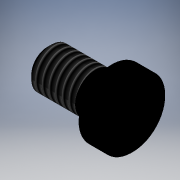
# Autodesk Inventor part: 25-2750-6
Saved by Autodesk Inventor 2017.3 (Build 213256000, 256)
## iProperties
Part Number: 25-2750-6
Material: Generic
Catalog Web Link: www.cadenas.de
Description: 25-2750_bolt-Socket Head Cap Screws
Vendor: 8020
Document SubType Name: Modeling
Designer: partserver
Manufacturer: 8020
Mass: 0.502109 g
Surface Area: 4.42769 cm^2
Volume: 0.502109 cm^3
Density: 1 g/cm^3
Appearance: PSOLRGB-0-0-0
Category: PARTsolutions
Company: 8020
Title: 25-2750-6
Author: Cadenas PARTsolutions
Comments: Socket Head Cap Screws
PSOL_IDENT_0: {$CADENAS_DATA\23d-libs\8020\metric\linear_motion\25_2750_bolt.prj},164 {VTYP=3D},{NB=25-2750-6},{LI
PSOL_IDENT_1: NA=25-2750-6},{NN=25-2750_bolt},{DATE=31.07.2020 09:21:29},{GEOMDATE=15.03.2012 10:20:00},{VERSION=}
PSOL_IDENT_2: ,{LINEID=60},{WBVAR=},{WBNUMERIC=}  {NB=25-2750-6},{LINA=25-2750-6},{KT=DUMMY},{PN=25-2750-6},{THRD=
PSOL_IDENT_3: M6 x 1.00},{THRD1=6.0000},{FIN=Black Zinc},{L=9.525},{TT=UNC},{A=10.000},{H=3.226},{J=3.17500},{T=1.
PSOL_IDENT_4: 613},{TH=6.0000},{NT=25-3204},{NO=1}
NB: 25-2750-6
NN: 25-2750_bolt
NT: 25-3204
NBSYN: $PN.
LINA: 25-2750-6
CATALOG: 80/20
PN: 25-2750-6
THRD: M6 x 1.00
FIN: Black Zinc
L: 9.525
H: 3.226
TH: 6
NO: 1
SUPPLIER: 8020
ARTICLENO: 25-2750-6
BOMINFO: 25-2750-6
CREATOR: CADENAS GmbH
Autodesk Inventor part; units mm, degrees
ref_plane "YZ Plane" through (0, 0, 0) normal (1, 0, 0) x (0, 1, 0)
ref_plane "XZ Plane" through (0, 0, 0) normal (0, 1, 0) x (-1, 0, 0)
ref_plane "XY Plane" through (0, 0, 0) normal (0, 0, 1) x (1, 0, 0)
sketch "Sketch_1" plane through (0, 0, 0) normal (0, 0, 1) x (1, 0, 0)
  line L0 (9.525, 0) -> (-3.226, 0)
  line L1 (-3.226, 0) -> (-3.226, 4.8476)
  line L2 (-3.226, 4.8476) -> (-3.0736, 5)
  line L3 (-3.0736, 5) -> (-0.254, 5)
  arc A0 (0, 4.746) -> (-0.254, 5) centre (-0.254, 4.746) ccw
  line L4 (0, 4.746) -> (0, 3.0762)
  arc A1 (0, 3.0762) -> (0.0762, 3) centre (0.0762, 3.0762) ccw
  line L5 (0.0762, 3) -> (8.9115, 3)
  line L6 (8.9115, 3) -> (9.525, 2.3865)
  line L7 (9.525, 2.3865) -> (9.525, 0)
  line L8 (9.525, 0) -> (-3.226, 0)
  constraints: 18 end point, 4 point on circle, 2 centre point
revolve "Revolution1" add sketch "Sketch_1" angle 360 about axis through (9.525, 0, 0) along (1, 0, 0)
thread "Thread1" size "M6x1" class "6g" standard "ISO Metric profile" length 6.5302
sketch "Sketch_3" plane through (-3.226, 0, 0) normal (1, 0, 0) x (0, 0, -1)
  line L0 (-1.5875, -0.9165) -> (0, -1.8331)
  line L1 (0, -1.8331) -> (1.5875, -0.9165)
  line L2 (1.5875, -0.9165) -> (1.5875, 0.9165)
  line L3 (1.5875, 0.9165) -> (0, 1.8331)
  line L4 (0, 1.8331) -> (-1.5875, 0.9165)
  line L5 (-1.5875, 0.9165) -> (-1.5875, -0.9165)
  constraints: 12 end point
extrude "Extrusion1" cut sketch "Sketch_3" along normal blind 1.613
sketch "Sketch_4" plane through (0, 0, 0) normal (0, 0, 1) x (1, 0, 0)
  line L0 (-0.6965, 0) -> (-1.613, 0)
  line L1 (-1.613, 0) -> (-1.613, 1.5875)
  line L2 (-1.613, 1.5875) -> (-0.6965, 0)
  line L3 (-0.6965, 0) -> (-1.613, 0)
  constraints: 8 end point
revolve "Revolution2" cut sketch "Sketch_4" angle 360 about axis through (-0.6965, 0, 0) along (1, 0, 0)
ref_plane "screw_XY" through (0, 0, 0) normal (1, 0, 0) x (0, 0, -1)
ref_plane "screw_YZ" through (0, 0, 0) normal (0, 0, -1) x (0, 1, 0)
ref_plane "screw_ZX" through (0, 0, 0) normal (0, 1, 0) x (1, 0, 0)
ref_plane "screw1_XY" through (9.525, 0, 0) normal (1, 0, 0) x (0, 0, -1)
ref_plane "screw1_YZ" through (9.525, 0, 0) normal (0, 0, -1) x (0, 1, 0)
ref_plane "screw1_ZX" through (9.525, 0, 0) normal (0, 1, 0) x (1, 0, 0)
ref_plane "screw2_XY" through (9.325, 0, 0) normal (1, 0, 0) x (0, 0, -1)
ref_plane "screw2_YZ" through (9.325, 0, 0) normal (0, 0, -1) x (0, 1, 0)
ref_plane "screw2_ZX" through (9.325, 0, 0) normal (0, 1, 0) x (1, 0, 0)
ref_plane "to_tnut_XY" through (0.29, 0, 0) normal (1, 0, 0) x (0, 0, -1)
ref_plane "to_tnut_YZ" through (0.29, 0, 0) normal (0, 0, -1) x (0, 1, 0)
ref_plane "to_tnut_ZX" through (0.29, 0, 0) normal (0, 1, 0) x (1, 0, 0)
body "Solid1"
